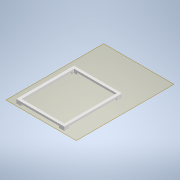
# Autodesk Inventor part: display_holder
Saved by Autodesk Inventor 2022 (Build 260153000, 153)
## iProperties
Created: 2021-12-06
Part Number: display_holder
Material: Generic
Document SubType Name: Modeling
Designer: simen
Density: 1 g/cm^3
Appearance: Default
Author: simen
## iProperties of the stored document display_holder_3DPrint.ipt
Created: 2021-12-08
Part Number: display_holder_3DPrint
Material: Generic
Document SubType Name: Modeling
Designer: simen
Density: 1 g/cm^3
Appearance: Default
Author: simen
Autodesk Inventor part; units mm, degrees
ref_plane "YZ Plane" through (0, 0, 0) normal (1, 0, 0) x (0, 1, 0)
ref_plane "XZ Plane" through (0, 0, 0) normal (0, 1, 0) x (-1, 0, 0)
ref_plane "XY Plane" through (0, 0, 0) normal (0, 0, 1) x (1, 0, 0)
ref_plane "Work Plane1" through (-15.1761, -6.8152, -116.1136) normal (0, 1, 0) x (0, 0, -1)
sketch "Sketch6" plane through (-15.1761, -6.8152, -116.1136) normal (0, 1, 0) x (0, 0, -1)
  line L0 (-99.3115, -54.3271) -> (-99.3115, -0.3271)
  line L1 (-34.3115, -0.3271) -> (-34.3115, -54.3271)
  line L2 (-99.3115, -0.3271) -> (-34.3115, -0.3271)
  line L3 (-99.3115, -54.3271) -> (-34.3115, -54.3271)
  line L4 (-96.3115, -3.3271) -> (-96.3115, -51.3271)
  line L5 (-96.3115, -51.3271) -> (-37.3115, -51.3271)
  line L6 (-37.3115, -51.3271) -> (-37.3115, -3.3271)
  line L7 (-37.3115, -3.3271) -> (-96.3115, -3.3271)
  line L8 (-79.0939, -0.3271) -> (-43.1029, -0.3271)
  line L9 (-43.1029, -3.3271) -> (-79.0939, -3.3271)
  point P0 (-116.1136, -15.1761)
  dimension "d19" = 54
  dimension "d27" = 65
  dimension "d36" = 3
  constraints: 20 end point, 3 horizontal, 2 perpendicular, 2 point on line, 1 parallel, 3 other
  measures "d19" distance of L1.start L1.end
  measures "d27" distance between parallel lines of L1 L0
  measures "d36" distance between parallel lines of L0 L4
extrude "Extrusion6" add sketch "Sketch6" along normal blind 4.2
sketch "Sketch7" plane through (-15.1761, -2.6152, -116.1136) normal (0, 1, 0) x (1, 0, 0)
  line L0 (54.3271, -34.3115) -> (0.3271, -34.3115) projected
  line L1 (0.3271, -99.3115) -> (54.3271, -99.3115) projected
  line L2 (0.3271, -99.3115) -> (54.3271, -99.3115) projected
  line L3 (1.3271, -99.3115) -> (1.3271, -94.3115)
  line L4 (-1.6729, -37.3115) -> (-1.6729, -34.3115)
  line L5 (56.3271, -99.3115) -> (56.3271, -81.4323)
  line L6 (55.9345, -81.4323) -> (51.9345, -81.4323) projected
  line L7 (51.9345, -49.4323) -> (55.9345, -49.4323) projected
  line L8 (54.9345, -49.4323) -> (54.9345, -34.3115)
  line L9 (0.3271, -34.3115) -> (0.3271, -99.3115) projected
  line L10 (54.3271, -99.3115) -> (54.3271, -34.3115) projected
  point P0 (15.1761, -116.1136)
  point P1 (54.9345, -86.4323)
  constraints: 8 end point, 6 point on line, 2 perpendicular, 1 parallel
extrude "Extrusion7" [suppressed]
sketch "Sketch8" plane through (-15.1761, -6.8152, -116.1136) normal (0, -1, 0) x (1, 0, 0)
  line L0 (54.3271, 99.3115) -> (54.3271, 34.3115) projected
  line L1 (54.3271, 34.3115) -> (0.3271, 34.3115) projected
  line L2 (0.3271, 34.3115) -> (0.3271, 99.3115) projected
  line L3 (0.3271, 99.3115) -> (54.3271, 99.3115) projected
  line L4 (3.3271, 37.3115) -> (51.3271, 37.3115) projected
  line L5 (51.3271, 37.3115) -> (51.3271, 96.3115) projected
  line L6 (51.3271, 96.3115) -> (3.3271, 96.3115) projected
  line L7 (3.3271, 96.3115) -> (3.3271, 37.3115) projected
  line L8 (3.3271, 96.3115) -> (3.3271, 37.3115) projected
  line L9 (3.3271, 93.1737) -> (0.3271, 93.1737)
  line L10 (3.3271, 96.3115) -> (3.3271, 37.3115) projected
  line L11 (3.3271, 39.3032) -> (0.3271, 39.3032)
  line L12 (0.3271, 34.3115) -> (0.3271, 99.3115) projected
  line L13 (3.3271, 37.3115) -> (51.3271, 37.3115) projected
  line L14 (6.5072, 37.3115) -> (6.5072, 34.3115)
  line L15 (54.3271, 34.3115) -> (0.3271, 34.3115) projected
  line L16 (3.3271, 37.3115) -> (51.3271, 37.3115) projected
  line L17 (49.2125, 37.3115) -> (49.2125, 34.3115)
  line L18 (54.3271, 34.3115) -> (0.3271, 34.3115) projected
  line L19 (51.3271, 37.3115) -> (51.3271, 96.3115) projected
  line L20 (51.3271, 39.7524) -> (54.3271, 39.7524)
  line L21 (54.3271, 99.3115) -> (54.3271, 34.3115) projected
  line L22 (51.3271, 94.1284) -> (54.3271, 94.1284)
  line L23 (51.3271, 96.3115) -> (3.3271, 96.3115) projected
  line L24 (48.2249, 96.3115) -> (48.2249, 99.3115)
  line L25 (0.3271, 99.3115) -> (54.3271, 99.3115) projected
  line L26 (6.0657, 96.3115) -> (6.0657, 99.3115)
  line L27 (51.3271, 96.3115) -> (3.3271, 96.3115) projected
  point P0 (15.1761, 116.1136)
  point P1 (49.2125, 37.3115)
  point P2 (6.5072, 37.3115)
  point P3 (0.3271, 39.3032)
  point P4 (3.3271, 39.3032)
  point P5 (3.3271, 93.1737)
  point P6 (6.0657, 99.3115)
  point P7 (48.2249, 96.3115)
  point P8 (48.2249, 99.3115)
  constraints: 16 end point, 16 point on line, 10 perpendicular
extrude "Extrusion8" cut sketch "Sketch8" against normal blind 2 contours L0 L20 L5 L22 | L24 L6 L26 L3 | L1 L14 L4 L17 | L9 L7 L11 L2
body "Solid2"
